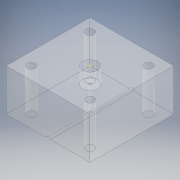
# Autodesk Inventor part: LS1_Aufsatz
Saved by Autodesk Inventor 2021 (Build 250183000, 183)
## iProperties
Created: 2021-05-21
Part Number: LS1_Aufsatz
Material: PMMA-Kunststoff
Document SubType Name: Modeling
Designer: Kauby
Density: 1.188 g/cm^3
Appearance: Polycarbonat - klar
Author: Kauby
Autodesk Inventor part; units mm, degrees
ref_plane "YZ Plane" through (0, 0, 0) normal (1, 0, 0) x (0, 1, 0)
ref_plane "XZ Plane" through (0, 0, 0) normal (0, 1, 0) x (-1, 0, 0)
ref_plane "XY Plane" through (0, 0, 0) normal (0, 0, 1) x (1, 0, 0)
sketch "Skizze1" plane through (0, 0, 0) normal (0, 1, 0) x (-1, 0, 0)
  line L0 (-15, 15) -> (15, 15)
  line L1 (15, 15) -> (15, -15)
  line L2 (15, -15) -> (-15, -15)
  line L3 (-15, -15) -> (-15, 15)
  line L4 (-15, 15) -> (15, -15) construction
  line L5 (15, 15) -> (-15, -15) construction
  point P0 (0, 0)
  dimension "d0" = 30
  dimension "d1" = 30
  constraints: 12 end point, 2 midpoint, 2 parallel, 1 horizontal, 1 perpendicular
  measures "d0" distance of L1.end L2.end
  measures "d1" distance of L0.end L1.end
extrude "Extrusion1" add sketch "Skizze1" along normal blind 15
sketch "Skizze2" plane through (-15, 0, 15) normal (0, 0, 1) x (1, 0, 0)
  circle A0 centre (15, 0) radius 0.8
  dimension "d4" = 1.6
  constraints: 1 centre point, 1 coincident
  measures "d4" diameter of A0
hole "Bohrung1" at (0, 0, 15) direction (0, 0, -1) diameter 1.6 end through all
sketch "Skizze3" plane through (0, 15, 0) normal (0, 1, 0) x (1, 0, 0)
  point P0 (0, 0)
hole "Bohrung2" at (0, 15, 0) direction (0, -1, 0) diameter 0.8 end through all
sketch "Skizze4" plane through (0, 15, 0) normal (0, 1, 0) x (1, 0, 0)
  point P0 (0, 0)
  point P1 (0, 0)
  constraints: 1 coincident
hole "Bohrung3" at (0, 15, 0) direction (0, -1, 0) diameter 5.5 depth 5.7
sketch "Skizze5" plane through (0, 15, 0) normal (0, 1, 0) x (1, 0, 0)
  point P0 (0, 0)
sketch "Skizze6" plane through (0, 15, 0) normal (0, 1, 0) x (1, 0, 0)
  line L0 (10.5, 10.5) -> (-10.5, 10.5)
  line L1 (-10.5, 10.5) -> (-10.5, -10.5)
  line L2 (-10.5, -10.5) -> (10.5, -10.5)
  line L3 (10.5, -10.5) -> (10.5, 10.5)
  circle A0 centre (0, 0) radius 0.4 projected
  line L4 (10.5, 10.5) -> (-10.5, -10.5) construction
  line L5 (-10.5, 10.5) -> (10.5, -10.5) construction
  dimension "d26" = 21
  dimension "d27" = 21
  constraints: 12 end point, 2 midpoint, 2 parallel, 1 horizontal, 1 perpendicular
  measures "d26" distance of L2.end L1.end
  measures "d27" distance of L1.end L0.end
hole "Bohrung4" at (10.5, 15, 10.5) at (-10.5, 15, 10.5) at (-10.5, 15, -10.5) at (10.5, 15, -10.5) direction (0, -1, 0) diameter 3 end through all
